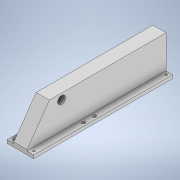
# Autodesk Inventor part: s_base2
Saved by Autodesk Inventor 2022 (Build 260153000, 153)
## iProperties
Created: 2021-08-20
Part Number: s_base2
Material: 一般
Document SubType Name: Modeling
Designer: yuta0
Density: 1 g/cm^3
Appearance: 既定
Author: yuta0
Autodesk Inventor part; units mm, degrees
ref_plane "YZ Plane" through (0, 0, 0) normal (1, 0, 0) x (0, 1, 0)
ref_plane "XZ Plane" through (0, 0, 0) normal (0, 1, 0) x (-1, 0, 0)
ref_plane "XY Plane" through (0, 0, 0) normal (0, 0, 1) x (1, 0, 0)
sketch "スケッチ1" plane through (0, 0, 0) normal (0, 0, 1) x (1, 0, 0)
  line L0 (-20, -2.5) -> (20, -2.5)
  line L1 (20, -2.5) -> (20, 2.5)
  line L2 (-20, 2.5) -> (-20, -2.5)
  line L3 (-20, -2.5) -> (20, 2.5) construction
  line L4 (20, -2.5) -> (-20, 2.5) construction
  line L5 (-10, 2.5) -> (10, 2.5)
  line L6 (10, 2.5) -> (10, 52.5)
  line L7 (10, 52.5) -> (-10, 52.5)
  line L8 (-10, 52.5) -> (-10, 2.5)
  line L9 (-10, 2.5) -> (10, 52.5) construction
  line L10 (10, 2.5) -> (-10, 52.5) construction
  line L11 (20, 2.5) -> (10, 2.5)
  line L12 (-10, 2.5) -> (-20, 2.5)
  point P0 (0, 0)
  point P1 (0, 27.5)
  point P2 (0, 27.5)
  point P3 (0, 0)
  dimension "d0" = 20
  dimension "d1" = 50
  dimension "d2" = 5
  dimension "d3" = 10
  constraints: 26 end point, 6 midpoint, 5 parallel, 2 horizontal, 2 perpendicular, 1 vertical alignment
  measures "d0" distance of L6.end L7.end
  measures "d1" distance of L5.end L6.end
  measures "d2" distance of L0.end L1.end
  measures "d3" distance between parallel lines of L8 L2
extrude "押し出し1" add sketch "スケッチ1" along normal mid plane 210
sketch "スケッチ4" plane through (20, -2.5, 105) normal (1, 0, 0) x (0, 0, -1)
  line L0 (0, 7) -> (33.61, 55)
  line L1 (210, 55) -> (0, 55) projected
  line L2 (0, 5) -> (0, 55) projected
  line L3 (210, 5) -> (0, 5) projected
  line L4 (210, 55) -> (210, 5) projected
  line L5 (0, 0) -> (0, 5) projected
  point P0 (105, 2.5)
  dimension "d18" = 35
  dimension "d21" = 2
  constraints: 2 end point, 2 point on line
  measures "d18" angle of L2 L0
  measures "d21" distance from line of L3 L0.start
extrude "押し出し3" cut sketch "スケッチ4" against normal through all contours L2 L1 L0
sketch "スケッチ6" plane through (10, 2.5, -105) normal (1, 0, 0) x (0, 0, -1)
  circle A0 centre (-158, 41) radius 6
  line L0 (0, 0) -> (-210, 0) projected
  line L1 (-210, -5) -> (-210, 0) projected
  point P0 (-105, -2.5)
  dimension "d33" = 12
  dimension "d34" = 41
  dimension "d35" = 52
  constraints: 1 centre point
  measures "d33" diameter of A0
  measures "d34" distance from line of L0 A0.centre
  measures "d35" distance from line of L1 A0.centre
extrude "押し出し4" cut sketch "スケッチ6" against normal through all
sketch "スケッチ7" plane through (10, 2.5, 105) normal (0, 1, 0) x (1, 0, 0)
  line L0 (0, 210) -> (10, 210) projected
  line L1 (10, 0) -> (0, 0) projected
  line L2 (-30, 210) -> (-30, 0) projected
  line L3 (-20, 0) -> (-30, 0) projected
  line L4 (-30, 210) -> (-20, 210) projected
  point P0 (-10, 105)
  point P1 (5, 5)
  point P2 (5, 79.86)
  point P3 (5, 96.483)
  point P4 (5, 205)
  point P5 (-25, 5)
  point P6 (-25, 79.86)
  point P7 (-25, 96.483)
  point P8 (-25, 205)
  dimension "d38" = 5
  dimension "d39" = 5
  dimension "d40" = 74.86
  dimension "d41" = 16.623
  dimension "d42" = 5
  dimension "d43" = 5
  dimension "d44" = 5
  dimension "d45" = 74.86
  dimension "d46" = 16.623
  measures "d38" distance from line of L0 point (5, 205)
  measures "d39" distance from line of L1 point (5, 5)
  measures "d40" distance of point (5, 79.86) point (5, 5)
  measures "d41" distance of point (5, 79.86) point (5, 96.483)
  measures "d42" distance from line of L2 point (-25, 5)
  measures "d43" distance from line of L3 point (-25, 5)
  measures "d44" distance from line of L4 point (-25, 205)
  measures "d45" distance of point (-25, 79.86) point (-25, 5)
  measures "d46" distance of point (-25, 96.483) point (-25, 79.86)
hole "穴3" at (15, 2.5, 100) at (15, 2.5, -100) at (-15, 2.5, 100) at (-15, 2.5, -100) direction (0, -1, 0) diameter 3.2 end through all
hole "穴4" at (15, 2.5, 25.14) at (15, 2.5, 8.517) at (-15, 2.5, 25.14) at (-15, 2.5, 8.517) direction (0, -1, 0) diameter 5.2 end through all
equation "\"d43\" = d39"
equation "\"d44\" = d38"
equation "\"d45\" = d40"
equation "\"d46\" = d41"
